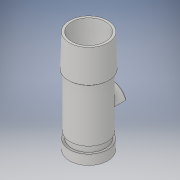
# Autodesk Inventor part: adaptadorDysonV3
Saved by Autodesk Inventor 2019.2 (Build 232265000, 265)
## iProperties
Created: 2018-11-03
Part Number: adaptadorDysonV3
Material: Generic
Document SubType Name: Modeling
Designer: garri
Density: 1 g/cm^3
Appearance: Default
Author: garri
## iProperties of the stored document adaptadorDyson_3DPrint.ipt
Created: 2018-11-03
Part Number: adaptadorDyson_3DPrint
Material: Generic
Document SubType Name: Modeling
Designer: garri
Density: 1 g/cm^3
Appearance: Default
Author: garri
Autodesk Inventor part; units mm, degrees
ref_plane "YZ Plane" through (0, 0, 0) normal (1, 0, 0) x (0, 1, 0)
ref_plane "XZ Plane" through (0, 0, 0) normal (0, 1, 0) x (-1, 0, 0)
sketch "Sketch1" plane through (0, 0, 0) normal (0, 1, 0) x (-1, 0, 0)
  circle A0 centre (0, 0) radius 14.75
  circle A1 centre (0, 0) radius 17.5
  dimension "d0" = 29.5
  dimension "d1" = 35
  constraints: 2 centre point, 2 coincident
  measures "d0" diameter of A0
  measures "d1" diameter of A1
extrude "Extrusion1" add sketch "Sketch1" along normal blind 9
sketch "Sketch2" plane through (0, 9, 0) normal (0, 1, 0) x (1, 0, 0)
  circle A0 centre (0, 0) radius 15.5
  circle A1 centre (0, 0) radius 14.75
  dimension "d4" = 31
  constraints: 2 centre point, 2 coincident
  measures "d4" diameter of A0
extrude "Extrusion2" add sketch "Sketch2" along normal blind 5
sketch "Sketch3" plane through (0, 14, 0) normal (0, 1, 0) x (1, 0, 0)
  circle A0 centre (0, 0) radius 14.75
  circle A1 centre (0, 0) radius 17
  constraints: 2 centre point, 2 coincident
extrude "Extrusion3" add sketch "Sketch3" along normal blind 50
fillet "Fillet1" radius 1 1 edges at (-17, 14, 0)
ref_plane "Work Plane1" through (0, 14, -17) normal (0, 0, 1) x (1, 0, 0)
sketch "Sketch4" plane through (0, 14, -17) normal (0, 0, 1) x (1, 0, 0)
  line L0 (21.7027, 23) -> (-22.3456, 23) construction
  line L1 (-17.5, -14) -> (17.5, -14) projected
  line L2 (0.0317, 23) -> (-1.25, 23)
  line L3 (0.0317, 23) -> (1.3134, 23)
  line L4 (1.3134, 33) -> (-1.25, 33)
  line L5 (0.0317, 23) -> (1.3134, 23)
  line L6 (0.0317, 23) -> (-1.25, 23)
  arc A0 (12.5317, 23) -> (-12.4683, 23) centre (0.0317, 9.875) ccw
  line L7 (12.5317, 23) -> (14.5317, 23)
  line L8 (-12.4683, 23) -> (-14.4683, 23)
  arc A1 (14.5317, 23) -> (-14.4683, 23) centre (0.0317, 17.4875) ccw
  line L9 (1.3134, 23) -> (1.3134, 27.9546)
  line L10 (1.3134, 32.947) -> (1.3134, 33)
  line L11 (-1.25, 23) -> (-1.25, 27.9546)
  line L12 (-1.25, 32.947) -> (-1.25, 33)
  line L13 (1.3134, 23) -> (-1.25, 23)
  line L14 (14.5317, 23) -> (12.5317, 23)
  line L15 (-12.4683, 23) -> (-14.4683, 23)
  point P0 (0, -14)
  point P1 (0.0317, 33)
  dimension "d10" = 37
  dimension "d16" = 10
  dimension "d17" = 12.5
  dimension "d18" = 12.5
  dimension "d19" = 5
  dimension "d20" = 2
  dimension "d21" = 2
  dimension "d22" = 44.0483
  constraints: 30 end point, 9 point on circle, 5 point on line, 4 horizontal, 4 perpendicular, 2 centre point, 1 collinear, 1 midpoint, 1 parallel
  measures "d10" distance between parallel lines of L1 L0
  measures "d16" distance of L3.end L4.start
  measures "d17" distance of L2.start L7.start
  measures "d18" distance of L2.start L8.start
  measures "d19" distance edge to line of A0 L0
  measures "d20" distance of L7.start L7.end
  measures "d21" distance of L8.start L8.end
  measures "d22" distance of L0.start L0.end
extrude "Extrusion4" add sketch "Sketch4" along normal blind 10 and the other way blind 4 contours L2 L11 A0 L9 L3 | A0 L8 A1 L7
chamfer "Chamfer1" distance 1.5 angle 45 1 edges at (0.0317, 47, -21)
sketch "Sketch5" plane through (0, 14, -21) normal (0, 0, -1) x (-1, 0, 0)
  line L0 (-1.3134, 27.9546) -> (-1.3134, 23) projected
  line L1 (-1.3134, 23) -> (-1.3134, 27.9546)
  arc A0 (12.4683, 23) -> (1.25, 27.9546) centre (-0.0317, 9.875) ccw projected
  line L2 (-1.3134, 27.9546) -> (1.25, 27.9546)
  line L3 (-1.3134, 23) -> (1.25, 23) projected
  line L4 (1.25, 27.9546) -> (1.25, 23)
  line L5 (1.25, 23) -> (-1.3134, 23)
  point P0 (0, -14)
  constraints: 8 end point, 2 collinear, 2 perpendicular
extrude "Extrusion5" cut sketch "Sketch5" against normal blind 1.5
sketch "Sketch6" plane through (0, 64, 0) normal (0, 1, 0) x (1, 0, 0)
  circle A0 centre (0, 0) radius 18.5
  circle A1 centre (0, 0) radius 15.5929
  dimension "d32" = 37
  constraints: 2 centre point, 2 coincident
  measures "d32" diameter of A0
extrude "Extrusion6" add sketch "Sketch6" along normal blind 30
chamfer "Chamfer3" distance 0.5 angle 45 1 edges at (-18.5, 64, 0)
sketch "Sketch9" plane through (0, 0, 0) normal (0, -1, 0) x (1, 0, 0)
  circle A0 centre (0, 0) radius 14.75
  constraints: 1 centre point, 1 coincident
extrude "Extrusion7" cut sketch "Sketch9" against normal through all
draft "FaceDraft4" angle 1.5 pull direction (0, 1, 0) faces at (15.5423, 84, 1.2547) (18.44, 84.1667, 1.4886) fixed edges at (-15.5929, 94, 0) (-18.5, 64.5, 0)
body "Solid1"
